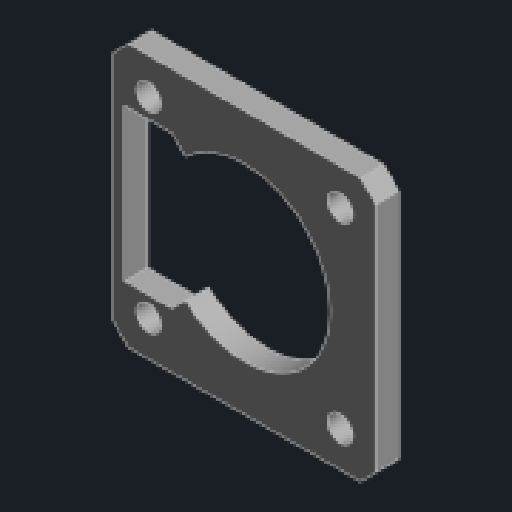
# Autodesk Inventor part: ArmEncoderSpacer
Saved by Autodesk Inventor 2023 (Build 270158000, 158)
## iProperties
Created: 2024-03-09
Part Number: ArmEncoderSpacer
Material: Generic
Document SubType Name: Modeling
Designer: valer
Density: 1 g/cm^3
Appearance: Default
Author: valer
Autodesk Inventor part; units mm, degrees
ref_plane "YZ Plane" through (0, 0, 0) normal (1, 0, 0) x (0, 1, 0)
ref_plane "XZ Plane" through (0, 0, 0) normal (0, 1, 0) x (-1, 0, 0)
ref_plane "XY Plane" through (0, 0, 0) normal (0, 0, 1) x (1, 0, 0)
sketch "Sketch1" plane through (0, 0, 0) normal (0, 0, 1) x (1, 0, 0)
  circle A0 centre (-10.3744, 12.3744) radius 1.621 projected
  circle A1 centre (14.3744, 12.3744) radius 1.621 projected
  circle A2 centre (14.3743, -12.3743) radius 1.6234 projected
  circle A3 centre (-10.3742, -12.3743) radius 1.6233 projected
  line L0 (-8.0786, 9.12) -> (-12.7986, 9.12) construction
  line L1 (-19, -24.05) -> (-21, -22.05) construction
  line L2 (19, -24.05) -> (-19, -24.05) construction
  line L3 (21, -22.05) -> (19, -24.05) construction
  line L4 (21, 22.05) -> (21, -22.05) construction
  line L5 (19, 24.05) -> (21, 22.05) construction
  line L6 (19, 24.05) -> (-19, 24.05) construction
  line L7 (-21, 22.05) -> (-19, 24.05) construction
  line L8 (-21, -22.05) -> (-21, 22.05) construction
  circle A4 centre (2, 0) radius 11.075 projected
  circle A5 centre (14.3744, 12.3744) radius 1.621 projected
  circle A6 centre (-10.3744, 12.3744) radius 1.621 projected
  circle A7 centre (14.3744, -12.3744) radius 1.621 projected
  circle A8 centre (-10.3744, -12.3744) radius 1.621 projected
  line L9 (-12.7986, -9.12) -> (-8.0786, -9.12) construction
  line L10 (-7.3786, 9.82) -> (-15, 9.82)
  line L11 (17, 17) -> (-13, 17) projected
  line L12 (-13, 17) -> (-15, 15) projected
  line L13 (-15, 15) -> (-15, -15) projected
  line L14 (-15, -15) -> (-13, -17) projected
  line L15 (-13, -17) -> (17, -17) projected
  line L16 (17, -17) -> (19, -15) projected
  line L17 (19, -15) -> (19, 15) projected
  line L18 (19, 15) -> (17, 17) projected
  line L19 (-15, -9.82) -> (-7.3786, -9.82)
  line L20 (-7.3786, -9.82) -> (-7.3786, 9.82) construction
  line L21 (-7.3786, 9.82) -> (-5.6074, 8.0488)
  line L22 (-7.3786, -9.82) -> (-5.6074, -8.0488)
  line L23 (-13.4986, 9.82) -> (-13.4986, -9.82)
  point P0 (0, 0)
  dimension "d0" = 0.7
  dimension "d1" = 0.7
  dimension "d2" = 0.7
  dimension "d3" = 45
  dimension "d4" = 45
  dimension "d7" = 0.7
  constraints: 12 end point, 4 point on line, 2 horizontal, 2 perpendicular, 2 point on circle
  measures "d0" horizontal distance of L10.start L0.start
  measures "d1" distance from line of L19 L9.end
  measures "d2" horizontal distance of L10.start L0.start
  measures "d3" angle of L21 L20
  measures "d4" angle of L22 L20
  measures "d7" horizontal distance of L23.start L0.end
extrude "Extrusion1" add sketch "Sketch1" against normal blind 5.05 contours A4 L21 L10 L13 L12 L11 L18 L17 L16 L15 L14 L19 L22 | L23 L19 L13 L10
body "Solid1"
